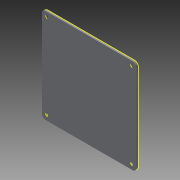
# Autodesk Inventor part: logo e-laska 2
Saved by Autodesk Inventor 2014 (Build 180170000, 170)
## iProperties
Created: 2017-04-19
Part Number: logo e-laska 2
Material: Ogólny
Document SubType Name: Modeling
Designer: hpdc7700
Density: 1 g/cm^3
Appearance: Domyślna
Author: hpdc7700
Autodesk Inventor part; units mm, degrees
ref_plane "YZ Plane" through (0, 0, 0) normal (1, 0, 0) x (0, 1, 0)
ref_plane "XZ Plane" through (0, 0, 0) normal (0, 1, 0) x (-1, 0, 0)
ref_plane "XY Plane" through (0, 0, 0) normal (0, 0, 1) x (1, 0, 0)
sketch "Szkic1" plane through (0, 0, 0) normal (0, 1, 0) x (-1, 0, 0)
  line L0 (-50, -50) -> (50, -50)
  line L1 (50, -50) -> (50, 50)
  line L2 (50, 50) -> (-50, 50)
  line L3 (-50, 50) -> (-50, -50)
  line L4 (-50, -50) -> (50, 50) construction
  line L5 (50, -50) -> (-50, 50) construction
  point P0 (0, 0)
  dimension "d0" = 100
  dimension "d1" = 100
  constraints: 12 end point, 2 midpoint, 2 parallel, 1 horizontal, 1 perpendicular
  measures "d0" distance of L2.end L1.end
  measures "d1" distance of L1.end L0.end
extrude "Wyciągnięcie proste1" add sketch "Szkic1" along normal blind 2
sketch "Szkic2" plane through (0, 2, 0) normal (0, 1, 0) x (1, 0, 0)
  line L0 (-45, -45) -> (45, -45)
  line L1 (45, -45) -> (45, 45)
  line L2 (45, 45) -> (-45, 45)
  line L3 (-45, 45) -> (-45, -45)
  line L4 (-45, -45) -> (45, 45) construction
  line L5 (45, -45) -> (-45, 45) construction
  circle A0 centre (-45, 45) radius 1.5
  circle A1 centre (-45, -45) radius 1.5
  circle A2 centre (45, -45) radius 1.5
  circle A3 centre (45, 45) radius 1.5
  point P0 (0, 0)
  dimension "d4" = 90
  dimension "d5" = 90
  dimension "d6" = 3
  dimension "d7" = 3
  dimension "d8" = 3
  dimension "d9" = 3
  constraints: 12 end point, 4 centre point, 4 coincident, 2 midpoint, 2 parallel, 1 horizontal, 1 perpendicular
  measures "d4" distance of L2.end L1.end
  measures "d5" distance of L1.end L0.end
  measures "d6" diameter of A0
  measures "d7" diameter of A1
  measures "d8" diameter of A2
  measures "d9" diameter of A3
extrude "Wyciągnięcie proste2" cut sketch "Szkic2" against normal blind 3 contours L3 A1 L0 | L0 A1 L3 | A2 L1 L0 | L0 L1 A2 | A0 L2 L3 | L3 L2 A0 | A3 L2 L1 | L1 L2 A3
chamfer "Faza1" distance 2 angle 45 4 edges at (-46.5, 2, 45) (-46.5, 2, -45) (43.5, 2, -45) (43.5, 2, 45)
fillet "Zaokrąglenie1" radius 4 4 edges at (50, 1, -50) (50, 1, 50) (-50, 1, 50) (-50, 1, -50)
sketch "Szkic3" plane through (0, 2, 0) normal (0, 1, 0) x (1, 0, 0)
  circle A0 centre (45, 45) radius 3.5 projected
  circle A1 centre (-45, -45) radius 3.5 projected
  arc A2 (-46, 50) -> (-50, 46) centre (-46, 46) ccw projected
  line L0 (-50, 46) -> (-50, -46) projected
  arc A3 (-50, -46) -> (-46, -50) centre (-46, -46) ccw projected
  line L1 (-46, -50) -> (46, -50) projected
  arc A4 (46, -50) -> (50, -46) centre (46, -46) ccw projected
  line L2 (50, -46) -> (50, 46) projected
  arc A5 (50, 46) -> (46, 50) centre (46, 46) ccw projected
  line L3 (46, 50) -> (-46, 50) projected
  circle A6 centre (-45, 45) radius 3.5 projected
  circle A7 centre (45, -45) radius 3.5 projected
  point P0 (0, 0)
equation "\"d10\" = d8"
